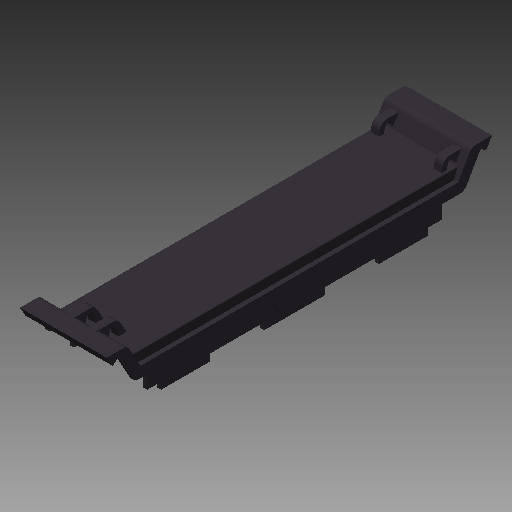
# Autodesk Inventor part: CH20M22 F BK 2418640000
Saved by Autodesk Inventor 2019.3 (Build 233278000, 278)
## iProperties
Category: PARTsolutions
Company: WEIDMUELLER
Created: 2018-11-15
Part Number: CH20M22 F BK 2418640000
Material: Generic
Catalog Web Link: www.cadenas.de
Description: CH20M22 F-Electronics housings
Vendor: WEIDMUELLER
Document SubType Name: Modeling
Designer: psadmin
Manufacturer: WEIDMUELLER
Mass: 4.43159 g
Surface Area: 91.1114 cm^2
Volume: 4.43159 cm^3
Density: 1 g/cm^3
Appearance: PSOLRGB-68-61-68
PSOL_IDENT_0: {$CADENAS_DATA\23d-libs\weidmueller\elektronikgehaeuse\einbaugehaeuse\ch20m\einzelteile\ch20m22-5\ch
PSOL_IDENT_1: 20m22-f.prj},189 {VTYP=3D},{NB=CH20M22 F BK 2418640000},{LINA=CH20M22 F BK 2418640000},{NN=CH20M22 F
PSOL_IDENT_2: },{DATE=31.03.2017 09:22:38},{GEOMDATE=16.09.2014 10:00:00},{VERSION=},{LINEID=10},{WBVAR=},{WBNUMER
PSOL_IDENT_3: IC=}  {NB=CH20M22 F BK 2418640000},{LINA=CH20M22 F BK 2418640000},{KT=DUMMY},{BEST=2418640000},{BZ=C
PSOL_IDENT_4: H20M22 F BK},{F=schwarz},{FCODE=0.27,0.24,0.27,0.00}
NN: CH20M22 F
NT: Electronics housings
NB: CH20M22 F BK 2418640000
NBSYN: $BZ. $BEST.
LINA: CH20M22 F BK 2418640000
BEST: 2418640000
BZ: CH20M22 F BK
F: black
SUPPLIER: WEIDMUELLER
ARTICLENO: CH20M22 F BK 2418640000
BOMINFO: CH20M22 F BK 2418640000
CREATOR: CADENAS GmbH
Title: CH20M22 F BK 2418640000
Author: Cadenas PARTsolutions
Comments: Electronics housings
Autodesk Inventor part; units mm, degrees
sketch "Sketch_1" plane through (0, 0, 0) normal (1, 0, 0) x (0, 1, 0)
  line L0 (9, 50) -> (6.6334, 48.6746)
  arc A0 (6.6334, 48.6746) -> (6.5448, 48.2266) centre (6.78, 48.4129) ccw
  line L1 (6.5448, 48.2266) -> (7.1155, 47.5061)
  arc A1 (6.9679, 46.7594) -> (7.1155, 47.5061) centre (6.7236, 47.1957) ccw
  line L2 (6.9679, 46.7594) -> (1.0228, 43.43)
  arc A2 (1.0228, 43.43) -> (0, 41.685) centre (2, 41.685) ccw
  line L3 (0, 41.685) -> (0, 2.5)
  line L4 (0, 2.5) -> (-2, 1.5674)
  line L5 (-2, 1.5674) -> (-2, -1.5674)
  line L6 (-2, -1.5674) -> (0, -2.5)
  line L7 (0, -2.5) -> (0, -41.685)
  arc A3 (0, -41.685) -> (1.0228, -43.43) centre (2, -41.685) ccw
  line L8 (1.0228, -43.43) -> (6.9679, -46.7594)
  arc A4 (7.1155, -47.5061) -> (6.9679, -46.7594) centre (6.7236, -47.1957) ccw
  line L9 (7.1155, -47.5061) -> (6.5448, -48.2266)
  arc A5 (6.5448, -48.2266) -> (6.6334, -48.6746) centre (6.78, -48.4129) ccw
  line L10 (6.6334, -48.6746) -> (9, -50)
  line L11 (9, -50) -> (9, -45.714)
  arc A6 (9, -45.714) -> (8.1051, -44.1871) centre (7.25, -45.714) ccw
  line L12 (8.1051, -44.1871) -> (2.8, -41.2161)
  line L13 (2.8, -41.2161) -> (2.8, 41.2161)
  line L14 (2.8, 41.2161) -> (8.1051, 44.1871)
  arc A7 (8.1051, 44.1871) -> (9, 45.714) centre (7.25, 45.714) ccw
  line L15 (9, 45.714) -> (9, 50)
  constraints: 32 end point, 16 point on circle, 8 centre point
extrude "Extrusion1" add sketch "Sketch_1" along normal mid plane 22.5
sketch "Sketch_15" plane through (0, 0, 0) normal (1, 0, 0) x (0, 1, 0)
  line L0 (0, 6.6489) -> (-3, 5.25)
  line L1 (-3, 5.25) -> (-3, -5.25)
  line L2 (-3, -5.25) -> (0, -6.6489)
  line L3 (0, -6.6489) -> (0, 6.6489)
  constraints: 8 end point
extrude "Extrusion2" add sketch "Sketch_15" along normal blind 11.25
sketch "Sketch_2" plane through (0, 0, 0) normal (0, 0, 1) x (1, 0, 0)
  line L0 (-10.14, 2.8) -> (10.14, 2.8)
  line L1 (10.14, 2.8) -> (9.879, 4.7826)
  arc A0 (9.879, 4.7826) -> (9.6311, 5) centre (9.6311, 4.75) ccw
  line L2 (9.6311, 5) -> (-9.6311, 5)
  arc A1 (-9.6311, 5) -> (-9.879, 4.7826) centre (-9.6311, 4.75) ccw
  line L3 (-9.879, 4.7826) -> (-10.14, 2.8)
  constraints: 8 end point, 4 point on circle, 2 centre point
extrude "Extrusion3" add sketch "Sketch_2" along normal mid plane 86
sketch "Sketch_3" plane through (0, 0, 0) normal (1, 0, 0) x (0, 1, 0)
  line L0 (6.78, 48.4) -> (-3, 48.4)
  line L1 (-3, 48.4) -> (-3, -48.4)
  line L2 (-3, -48.4) -> (6.78, -48.4)
  line L3 (6.78, -48.4) -> (7.1588, -48.2985)
  arc A0 (7.1588, -48.2985) -> (7.9, -47.3326) centre (6.9, -47.3326) ccw
  line L4 (7.9, -47.3326) -> (7.9, -45.9023)
  arc A1 (7.9, -45.9023) -> (7.3886, -45.0298) centre (6.9, -45.9023) ccw
  line L5 (7.3886, -45.0298) -> (1.8, -41.9)
  line L6 (1.8, -41.9) -> (1.8, 41.9)
  line L7 (1.8, 41.9) -> (7.3886, 45.0298)
  arc A2 (7.3886, 45.0298) -> (7.9, 45.9023) centre (6.9, 45.9023) ccw
  line L8 (7.9, 45.9023) -> (7.9, 47.3326)
  arc A3 (7.9, 47.3326) -> (7.1588, 48.2985) centre (6.9, 47.3326) ccw
  line L9 (7.1588, 48.2985) -> (6.78, 48.4)
  constraints: 20 end point, 8 point on circle, 4 centre point
extrude "Extrusion4" cut sketch "Sketch_3" along normal mid plane 21.5
sketch "Sketch_4" plane through (0, 0, 0) normal (1, 0, 0) x (0, 1, 0)
  line L0 (6.78, 48.4) -> (-3, 48.4)
  line L1 (-3, 48.4) -> (-3, -48.4)
  line L2 (-3, -48.4) -> (6.78, -48.4)
  line L3 (6.78, -48.4) -> (7.1588, -48.2985)
  arc A0 (7.1588, -48.2985) -> (7.9, -47.3326) centre (6.9, -47.3326) ccw
  line L4 (7.9, -47.3326) -> (7.9, -45.9162)
  arc A1 (7.9, -45.9162) -> (7.3886, -45.0437) centre (6.9, -45.9162) ccw
  line L5 (7.3886, -45.0437) -> (3.9, -43.09)
  line L6 (3.9, -43.09) -> (3.9, 43.09)
  line L7 (3.9, 43.09) -> (7.3886, 45.0437)
  arc A2 (7.3886, 45.0437) -> (7.9, 45.9162) centre (6.9, 45.9162) ccw
  line L8 (7.9, 45.9162) -> (7.9, 47.3326)
  arc A3 (7.9, 47.3326) -> (7.1588, 48.2985) centre (6.9, 47.3326) ccw
  line L9 (7.1588, 48.2985) -> (6.78, 48.4)
  constraints: 20 end point, 8 point on circle, 4 centre point
extrude "Extrusion5" cut sketch "Sketch_4" along normal mid plane 18
sketch "Sketch_5" plane through (9, 0, 0) normal (1, 0, 0) x (0, 0, -1)
  line L0 (-38.25, -4.7) -> (-34.635, -4.7)
  line L1 (-34.635, -4.7) -> (-34.635, -6.5)
  line L2 (-34.635, -6.5) -> (-21.835, -6.5)
  line L3 (-21.835, -6.5) -> (-21.835, -4.7)
  line L4 (-21.835, -4.7) -> (-7.835, -4.7)
  line L5 (-7.835, -4.7) -> (-7.835, -6.5)
  line L6 (-7.835, -6.5) -> (7.835, -6.5)
  line L7 (7.835, -6.5) -> (7.835, -4.7)
  line L8 (7.835, -4.7) -> (21.835, -4.7)
  line L9 (21.835, -4.7) -> (21.835, -6.5)
  line L10 (21.835, -6.5) -> (34.635, -6.5)
  line L11 (34.635, -6.5) -> (34.635, -4.7)
  line L12 (34.635, -4.7) -> (38.25, -4.7)
  line L13 (38.25, -4.7) -> (38.25, 1.8)
  line L14 (38.25, 1.8) -> (-38.25, 1.8)
  line L15 (-38.25, 1.8) -> (-38.25, -4.7)
  constraints: 32 end point
extrude "Extrusion6" add sketch "Sketch_5" along normal blind 1
sketch "Sketch_6" plane through (-9, 0, 0) normal (1, 0, 0) x (0, 0, -1)
  line L0 (-38.25, -4.7) -> (-34.635, -4.7)
  line L1 (-34.635, -4.7) -> (-34.635, -6.5)
  line L2 (-34.635, -6.5) -> (-21.835, -6.5)
  line L3 (-21.835, -6.5) -> (-21.835, -4.7)
  line L4 (-21.835, -4.7) -> (-7.835, -4.7)
  line L5 (-7.835, -4.7) -> (-7.835, -6.5)
  line L6 (-7.835, -6.5) -> (7.835, -6.5)
  line L7 (7.835, -6.5) -> (7.835, -4.7)
  line L8 (7.835, -4.7) -> (21.835, -4.7)
  line L9 (21.835, -4.7) -> (21.835, -6.5)
  line L10 (21.835, -6.5) -> (34.635, -6.5)
  line L11 (34.635, -6.5) -> (34.635, -4.7)
  line L12 (34.635, -4.7) -> (38.25, -4.7)
  line L13 (38.25, -4.7) -> (38.25, 1.8)
  line L14 (38.25, 1.8) -> (-38.25, 1.8)
  line L15 (-38.25, 1.8) -> (-38.25, -4.7)
  constraints: 32 end point
extrude "Extrusion7" add sketch "Sketch_6" against normal blind 1
sketch "Sketch_7" plane through (0, 3.9, 0) normal (0, 1, 0) x (1, 0, 0)
  arc A0 (3.75, -36.95) -> (3.75, -38.05) centre (3.75, -37.5) ccw
  line L0 (3.75, -38.05) -> (7.7, -38.05)
  arc A1 (7.7, -38.05) -> (7.7, -36.95) centre (7.7, -37.5) ccw
  line L1 (7.7, -36.95) -> (3.75, -36.95)
  constraints: 4 end point, 4 point on circle, 2 centre point
extrude "Extrusion8" add sketch "Sketch_7" against normal blind 4.25
sketch "Sketch_8" plane through (0, 3.9, 0) normal (0, 1, 0) x (1, 0, 0)
  arc A0 (3.75, 38.05) -> (3.75, 36.95) centre (3.75, 37.5) ccw
  line L0 (3.75, 36.95) -> (7.7, 36.95)
  arc A1 (7.7, 36.95) -> (7.7, 38.05) centre (7.7, 37.5) ccw
  line L1 (7.7, 38.05) -> (3.75, 38.05)
  constraints: 4 end point, 4 point on circle, 2 centre point
extrude "Extrusion9" add sketch "Sketch_8" against normal blind 4.25
sketch "Sketch_10" plane through (3, 0, 0) normal (1, 0, 0) x (0, 0, -1)
  line L0 (-45.75, 8.5) -> (-43, 5)
  line L1 (-43, 5) -> (-42.3681, 5)
  line L2 (-42.3681, 5) -> (-41.9848, 7.1736)
  arc A0 (-40.0152, 7.1736) -> (-41.9848, 7.1736) centre (-41, 7) ccw
  line L3 (-40.0152, 7.1736) -> (-39.6319, 5)
  line L4 (-39.6319, 5) -> (-37.5877, 5)
  line L5 (-37.5877, 5) -> (-39.255, 7.9772)
  arc A1 (-39.255, 7.9772) -> (-41, 9) centre (-41, 7) ccw
  line L6 (-41, 9) -> (-45.75, 9)
  line L7 (-45.75, 9) -> (-45.75, 8.5)
  constraints: 16 end point, 4 point on circle, 2 centre point
extrude "Extrusion10" add sketch "Sketch_10" along normal mid plane 2
sketch "Sketch_11" plane through (-3, 0, 0) normal (1, 0, 0) x (0, 0, -1)
  line L0 (-45.75, 8.5) -> (-43, 5)
  line L1 (-43, 5) -> (-42.3681, 5)
  line L2 (-42.3681, 5) -> (-41.9848, 7.1736)
  arc A0 (-40.0152, 7.1736) -> (-41.9848, 7.1736) centre (-41, 7) ccw
  line L3 (-40.0152, 7.1736) -> (-39.6319, 5)
  line L4 (-39.6319, 5) -> (-37.5877, 5)
  line L5 (-37.5877, 5) -> (-39.255, 7.9772)
  arc A1 (-39.255, 7.9772) -> (-41, 9) centre (-41, 7) ccw
  line L6 (-41, 9) -> (-45.75, 9)
  line L7 (-45.75, 9) -> (-45.75, 8.5)
  constraints: 16 end point, 4 point on circle, 2 centre point
extrude "Extrusion11" add sketch "Sketch_11" along normal mid plane 2
sketch "Sketch_12" plane through (8.165, 0, 0) normal (1, 0, 0) x (0, 0, -1)
  line L0 (39, 5) -> (40.245, 5)
  line L1 (40.245, 5) -> (40.5858, 6.2718)
  arc A0 (42.646, 6.0915) -> (40.5858, 6.2718) centre (41.6, 6) ccw
  line L2 (42.646, 6.0915) -> (42.7415, 5)
  line L3 (42.7415, 5) -> (43.2, 5)
  line L4 (43.2, 5) -> (44.2, 7.95)
  line L5 (44.2, 7.95) -> (41.1264, 7.95)
  arc A1 (41.1264, 7.95) -> (39.1403, 6.1851) centre (41.1264, 5.95) ccw
  line L6 (39.1403, 6.1851) -> (39, 5)
  constraints: 14 end point, 4 point on circle, 2 centre point
extrude "Extrusion12" add sketch "Sketch_12" along normal mid plane 2.09
sketch "Sketch_13" plane through (-8.165, 0, 0) normal (1, 0, 0) x (0, 0, -1)
  line L0 (39, 5) -> (40.245, 5)
  line L1 (40.245, 5) -> (40.5858, 6.2718)
  arc A0 (42.646, 6.0915) -> (40.5858, 6.2718) centre (41.6, 6) ccw
  line L2 (42.646, 6.0915) -> (42.7415, 5)
  line L3 (42.7415, 5) -> (43.2, 5)
  line L4 (43.2, 5) -> (44.2, 7.95)
  line L5 (44.2, 7.95) -> (41.1264, 7.95)
  arc A1 (41.1264, 7.95) -> (39.1403, 6.1851) centre (41.1264, 5.95) ccw
  line L6 (39.1403, 6.1851) -> (39, 5)
  constraints: 14 end point, 4 point on circle, 2 centre point
extrude "Extrusion13" add sketch "Sketch_13" along normal mid plane 2.09
ref_plane "CP_XY" through (0, 0, 0) normal (0, 1, 0) x (1, 0, 0)
ref_plane "CP_YZ" through (0, 0, 0) normal (1, 0, 0) x (0, 0, -1)
ref_plane "CP_ZX" through (0, 0, 0) normal (0, 0, -1) x (0, 1, 0)
ref_plane "mitCover_XY" through (0, 7, 41) normal (-1, 0, 0) x (0, 0, -1)
ref_plane "mitCover_YZ" through (0, 7, 41) normal (0, 0, -1) x (0, -1, 0)
ref_plane "mitCover_ZX" through (0, 7, 41) normal (0, -1, 0) x (-1, 0, 0)
body "Solid1"
